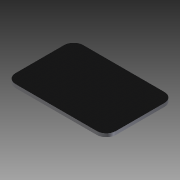
# Autodesk Inventor part: Tablet - Nexus 10
Saved by Autodesk Inventor 2014 (Build 180170000, 170)
## iProperties
Created: 2013-08-01
Part Number: Tablet - Nexus 10
Material: Allgemein
Document SubType Name: Modeling
Designer: vogel
Density: 1 g/cm^3
Appearance: Vorgabe
Author: vogel
Autodesk Inventor part; units mm, degrees
ref_plane "YZ Plane" through (0, 0, 0) normal (1, 0, 0) x (0, 1, 0)
ref_plane "XZ Plane" through (0, 0, 0) normal (0, 1, 0) x (-1, 0, 0)
ref_plane "XY Plane" through (0, 0, 0) normal (0, 0, 1) x (1, 0, 0)
sketch "Skizze1" plane through (0, 0, 0) normal (0, 0, 1) x (1, 0, 0)
  line L0 (-191.9087, 0) -> (191.9087, 0) projected
  line L1 (0, -131.7087) -> (0, 131.7087) projected
  line L2 (-106.9, 88.9) -> (106.9, 88.9)
  line L3 (131.9, 63.9) -> (131.9, -63.9)
  line L4 (106.9, -88.9) -> (-106.9, -88.9)
  line L5 (-131.9, -63.9) -> (-131.9, 63.9)
  arc A0 (-106.9, 88.9) -> (-131.9, 63.9) centre (-106.9, 63.9) ccw
  arc A1 (131.9, 63.9) -> (106.9, 88.9) centre (106.9, 63.9) ccw
  arc A2 (106.9, -88.9) -> (131.9, -63.9) centre (106.9, -63.9) ccw
  arc A3 (-131.9, -63.9) -> (-106.9, -88.9) centre (-106.9, -63.9) ccw
  point P0 (0, 0)
  point P1 (131.9, -88.9)
  point P2 (131.9, 88.9)
  dimension "d0" = 263.8
  dimension "d1" = 177.8
  dimension "d2" = 25
  constraints: 8 end point, 8 point on circle, 8 tangent, 4 centre point, 4 point on line, 3 equal radius, 2 parallel, 1 horizontal, 1 perpendicular, 2 other
  measures "d0" distance between parallel lines of L3 L5
  measures "d1" distance of point (131.9, 88.9) point (131.9, -88.9)
  measures "d2" radius of A0
extrude "Extrusion1" add sketch "Skizze1" along normal blind 8.9
